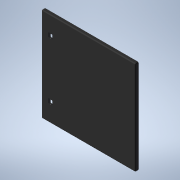
# Autodesk Inventor part: 155X_01_01(1)_P2
Saved by Autodesk Inventor 2021 (Build 250183000, 183)
## iProperties
Created: 2025-07-29
Part Number: 155X_01_01(1)_P2
Material: Generic
Catalog Web Link: www.cadenas.de
Description: AE 2.0 Einzeltuer-AE 2.0 Einzeltuer
Vendor: RITTAL
Document SubType Name: Modeling
Designer: psAdmin
Manufacturer: RITTAL
Mass: 530.122 g
Surface Area: 6232.6 cm^2
Volume: 530.122 cm^3
Density: 1 g/cm^3
Appearance: PSOLRGB-176-176-176
Category: PARTsolutions
Company: RITTAL
Title: 155X_01_01(1)_P2
Author: Cadenas PARTsolutions
Comments: AE 2.0 Einzeltuer
PSOL_IDENT_0: {$CADENAS_DATA/23d-libs/rittal/schaltschranksys/kompakt_schaltschr/parts_ae_2_0/einzeltuer_ae_2_0.pr
PSOL_IDENT_1: j},196 {VTYP=3D},{NB=155X_01_01(1)_P2},{LINA=155X_01_01(1)_P2},{NN=AE 2.0 Einzeltuer},{DATE=28.04.20
PSOL_IDENT_2: 25 21:11:31},{GEOMDATE=11.04.2025 11:21:47},{VERSION=},{LINEID=180},{WBVAR=DETAIL},{WBNUMERIC=DETAIL
PSOL_IDENT_3: }  {NB=155X_01_01(1)_P2},{LINA=155X_01_01(1)_P2},{KT=DUMMY},{BEST=155X},{DETAIL=1},{BEZ1=Neues Kompa
PSOL_IDENT_4: ktgehäuse},{BEZ2=Stahlblech},{BEZ3=eintürig},{B=500},{H=500},{VERS=1},{W=494},{W1=425},{W3=0},{HH=49
PSOL_IDENT_5: 4},{H1=375},{H2=440},{H4=58.0},{H5=300.000},{H6=350.000},{H7=350.000},{D=16.5},{ST=1.5},{R1=5.0},{GE
PSOL_IDENT_6: W=0},{CNSECLASS51=27-18-01-02},{CNSECLASS70=27-18-01-01},{CNSECLASS80=27-18-01-01},{CNSETIM40=EC0002
PSOL_IDENT_7: 61}
NB: 155X_01_01(1)_P2
NN: AE 2.0 Einzeltuer
NT: AE 2.0 Einzeltuer
NBSYN: $BEST._01_01($DETAIL.)_P2
LINA: 155X_01_01(1)_P2
CATALOG: Rittal
BEST: 155X
DETAIL: hoch
BEZ1: Neues Kompaktgehäuse
BEZ2: Stahlblech
BEZ3: eintürig
B: 500
H: 500
VERS: 1
W: 494
W1: 425
W3: 0
HH: 494
H1: 375
H2: 440
H4: 58
H5: 300
H6: 350
H7: 350
D: 16.5
ST: 1.5
R1: 5
GEW: 0
CNSECLASS70: 27-18-01-01
CNSECLASS80: 27-18-01-01
SUPPLIER: RITTAL
ARTICLENO: 155X_01_01(1)_P2
BOMINFO: 155X_01_01(1)_P2
CREATOR: CADENAS GmbH
Autodesk Inventor part; units mm, degrees
sketch "Sketch_1" plane through (0, 0, 0) normal (0, 1, 0) x (1, 0, 0)
  arc A0 (-247, 5) -> (-242, 0) centre (-242, 5) ccw
  line L0 (-242, 0) -> (242, 0)
  arc A1 (242, 0) -> (247, 5) centre (242, 5) ccw
  line L1 (247, 5) -> (247, 16.5)
  line L2 (247, 16.5) -> (245.5, 16.5)
  line L3 (245.5, 16.5) -> (245.5, 5)
  arc A2 (242, 1.5) -> (245.5, 5) centre (242, 5) ccw
  line L4 (242, 1.5) -> (-242, 1.5)
  arc A3 (-245.5, 5) -> (-242, 1.5) centre (-242, 5) ccw
  line L5 (-245.5, 5) -> (-245.5, 16.5)
  line L6 (-245.5, 16.5) -> (-247, 16.5)
  line L7 (-247, 16.5) -> (-247, 5)
  constraints: 16 end point, 8 point on circle, 4 centre point
extrude "Extrusion1" add sketch "Sketch_1" along normal mid plane 484
sketch "Sketch_3" plane through (0, 242, 0) normal (0, 1, 0) x (1, 0, 0)
  line L0 (242, 0) -> (242, 16.5)
  arc A0 (242, 1.5) -> (245.5, 5) centre (242, 5) ccw
  line L1 (245.5, 5) -> (245.5, 16.5)
  line L2 (245.5, 16.5) -> (247, 16.5)
  line L3 (247, 16.5) -> (247, 5)
  arc A1 (242, 0) -> (247, 5) centre (242, 5) ccw
  line L4 (242, 0) -> (242, 1.5)
  constraints: 10 end point, 4 point on circle, 2 centre point
revolve "Revolution1" add sketch "Sketch_3" angle 90 about axis through (242, 242, 0) along (0, 0, 1)
sketch "Sketch_4" plane through (0, 242, 0) normal (0, 1, 0) x (1, 0, 0)
  line L0 (-242, 16.5) -> (-242, 0)
  arc A0 (-247, 5) -> (-242, 0) centre (-242, 5) ccw
  line L1 (-247, 5) -> (-247, 16.5)
  line L2 (-247, 16.5) -> (-245.5, 16.5)
  line L3 (-245.5, 16.5) -> (-245.5, 5)
  arc A1 (-245.5, 5) -> (-242, 1.5) centre (-242, 5) ccw
  line L4 (-242, 1.5) -> (-242, 0)
  constraints: 10 end point, 4 point on circle, 2 centre point
revolve "Revolution2" add sketch "Sketch_4" angle 90 about axis through (-242, 242, -16.5) along (0, 0, -1)
sketch "Sketch_5" plane through (0, -242, 0) normal (0, 1, 0) x (1, 0, 0)
  line L0 (242, 0) -> (242, 16.5)
  arc A0 (242, 1.5) -> (245.5, 5) centre (242, 5) ccw
  line L1 (245.5, 5) -> (245.5, 16.5)
  line L2 (245.5, 16.5) -> (247, 16.5)
  line L3 (247, 16.5) -> (247, 5)
  arc A1 (242, 0) -> (247, 5) centre (242, 5) ccw
  line L4 (242, 0) -> (242, 1.5)
  constraints: 10 end point, 4 point on circle, 2 centre point
revolve "Revolution3" add sketch "Sketch_5" angle 90 about axis through (242, -242, 0) along (0, 0, -1)
sketch "Sketch_6" plane through (0, -242, 0) normal (0, 1, 0) x (1, 0, 0)
  line L0 (-242, 16.5) -> (-242, 0)
  arc A0 (-247, 5) -> (-242, 0) centre (-242, 5) ccw
  line L1 (-247, 5) -> (-247, 16.5)
  line L2 (-247, 16.5) -> (-245.5, 16.5)
  line L3 (-245.5, 16.5) -> (-245.5, 5)
  arc A1 (-245.5, 5) -> (-242, 1.5) centre (-242, 5) ccw
  line L4 (-242, 1.5) -> (-242, 0)
  constraints: 10 end point, 4 point on circle, 2 centre point
revolve "Revolution4" add sketch "Sketch_6" angle 90 about axis through (-242, -242, -16.5) along (0, 0, 1)
sketch "Sketch_2" plane through (0, 0, 0) normal (1, 0, 0) x (0, 0, -1)
  line L0 (0, 242) -> (0, -242)
  arc A0 (0, -242) -> (5, -247) centre (5, -242) ccw
  line L1 (5, -247) -> (16.5, -247)
  line L2 (16.5, -247) -> (16.5, -245.5)
  line L3 (16.5, -245.5) -> (5, -245.5)
  arc A1 (1.5, -242) -> (5, -245.5) centre (5, -242) ccw
  line L4 (1.5, -242) -> (1.5, 242)
  arc A2 (5, 245.5) -> (1.5, 242) centre (5, 242) ccw
  line L5 (5, 245.5) -> (16.5, 245.5)
  line L6 (16.5, 245.5) -> (16.5, 247)
  line L7 (16.5, 247) -> (5, 247)
  arc A3 (5, 247) -> (0, 242) centre (5, 242) ccw
  constraints: 16 end point, 8 point on circle, 4 centre point
extrude "Extrusion2" add sketch "Sketch_2" along normal mid plane 484
sketch "Sketch_44" plane through (231, 0, 0) normal (1, 0, 0) x (0, 0, -1)
  line L0 (1.5, -224.6934) -> (1.5, 224.6934)
  line L1 (1.5, 224.6934) -> (7.5, 224.6934)
  line L2 (7.5, 224.6934) -> (7, 208)
  line L3 (7, 208) -> (7, -208)
  line L4 (7, -208) -> (7.5, -224.6934)
  line L5 (7.5, -224.6934) -> (1.5, -224.6934)
  line L6 (1.5, -224.6934) -> (1.5, 224.6934)
  constraints: 14 end point
revolve "Revolution5" add sketch "Sketch_44" angle 180 mid plane about axis through (231, -224.6934, -1.5) along (0, 1, 0)
sketch "Sketch_45" plane through (0, 224.6934, 0) normal (0, 1, 0) x (1, 0, 0)
  line L0 (241, 7.5) -> (241, 1.5)
  line L1 (225, 1.5) -> (237, 1.5)
  arc A0 (237, 1.5) -> (225, 1.5) centre (231, 1.5) ccw
  constraints: 4 end point, 2 point on circle, 1 centre point
revolve "Revolution6" add sketch "Sketch_45" angle 39.715 about axis through (241, 224.6934, -7.5) along (0, 0, -1)
sketch "Sketch_47" plane through (0, 224.6934, 0) normal (0, 1, 0) x (1, 0, 0)
  line L0 (-241, 1.5) -> (-241, 7.5)
  line L1 (-237, 1.5) -> (-225, 1.5)
  arc A0 (-225, 1.5) -> (-237, 1.5) centre (-231, 1.5) ccw
  constraints: 4 end point, 2 point on circle, 1 centre point
revolve "Revolution7" add sketch "Sketch_47" angle 39.715 about axis through (-241, 224.6934, -1.5) along (0, 0, 1)
sketch "Sketch_46" plane through (241, 224.6934, 0) normal (-0.6389711, -0.7692308, 0) x (-0.7692308, 0.6389711, 0)
  line L0 (13, 6.6962) -> (13, 1.5)
  line L1 (13, 1.5) -> (4, 1.5)
  arc A0 (13, 6.6962) -> (4, 1.5) centre (10, 1.5) ccw
  line L2 (13, 6.6962) -> (13, 1.5)
  constraints: 6 end point, 2 point on circle, 1 centre point
revolve "Revolution8" add sketch "Sketch_46" angle 169.43 about axis through (231, 233, -6.6962) along (0, 0, 1)
sketch "Sketch_49" plane through (-241, 224.6934, 0) normal (-0.6389711, 0.7692308, 0) x (0.7692308, 0.6389711, 0)
  line L0 (13, 6.6962) -> (13, 1.5)
  line L1 (13, 1.5) -> (4, 1.5)
  arc A0 (13, 6.6962) -> (4, 1.5) centre (10, 1.5) ccw
  line L2 (13, 6.6962) -> (13, 1.5)
  constraints: 6 end point, 2 point on circle, 1 centre point
revolve "Revolution9" add sketch "Sketch_49" angle 169.43 about axis through (-231, 233, -6.6962) along (0, 0, -1)
sketch "Sketch_48" plane through (231, 233, 0) normal (-0.7692308, -0.6389711, 0) x (-0.6389711, 0.7692308, 0)
  line L0 (13, 7.5) -> (13, 1.5)
  line L1 (-3, 1.5) -> (9, 1.5)
  arc A0 (9, 1.5) -> (-3, 1.5) centre (3, 1.5) ccw
  constraints: 4 end point, 2 point on circle, 1 centre point
revolve "Revolution10" add sketch "Sketch_48" angle 39.715 about axis through (222.6934, 243, -7.5) along (0, 0, -1)
sketch "Sketch_50" plane through (-231, 233, 0) normal (-0.7692308, 0.6389711, 0) x (0.6389711, 0.7692308, 0)
  line L0 (13, 7.5) -> (13, 1.5)
  line L1 (-3, 1.5) -> (9, 1.5)
  arc A0 (9, 1.5) -> (-3, 1.5) centre (3, 1.5) ccw
  constraints: 4 end point, 2 point on circle, 1 centre point
revolve "Revolution11" add sketch "Sketch_50" angle 39.715 about axis through (-222.6934, 243, -7.5) along (0, 0, 1)
sketch "Sketch_51" plane through (-231, 0, 0) normal (1, 0, 0) x (0, 0, -1)
  line L0 (1.5, -224.6934) -> (1.5, 224.6934)
  line L1 (1.5, 224.6934) -> (7.5, 224.6934)
  line L2 (7.5, 224.6934) -> (7, 208)
  line L3 (7, 208) -> (7, -208)
  line L4 (7, -208) -> (7.5, -224.6934)
  line L5 (7.5, -224.6934) -> (1.5, -224.6934)
  line L6 (1.5, -224.6934) -> (1.5, 224.6934)
  constraints: 14 end point
revolve "Revolution12" add sketch "Sketch_51" angle 180 mid plane about axis through (-231, -224.6934, -1.5) along (0, 1, 0)
sketch "Sketch_52" plane through (0, -224.6934, 0) normal (0, 1, 0) x (1, 0, 0)
  line L0 (241, 7.5) -> (241, 1.5)
  line L1 (225, 1.5) -> (237, 1.5)
  arc A0 (237, 1.5) -> (225, 1.5) centre (231, 1.5) ccw
  constraints: 4 end point, 2 point on circle, 1 centre point
revolve "Revolution13" add sketch "Sketch_52" angle 39.715 about axis through (241, -224.6934, -7.5) along (0, 0, 1)
sketch "Sketch_53" plane through (0, -224.6934, 0) normal (0, 1, 0) x (1, 0, 0)
  line L0 (-241, 1.5) -> (-241, 7.5)
  line L1 (-237, 1.5) -> (-225, 1.5)
  arc A0 (-225, 1.5) -> (-237, 1.5) centre (-231, 1.5) ccw
  constraints: 4 end point, 2 point on circle, 1 centre point
revolve "Revolution14" add sketch "Sketch_53" angle 39.715 about axis through (-241, -224.6934, -1.5) along (0, 0, -1)
sketch "Sketch_54" plane through (241, -224.6934, 0) normal (0.6389711, -0.7692308, 0) x (-0.7692308, -0.6389711, 0)
  line L0 (13, 6.6962) -> (13, 1.5)
  line L1 (13, 1.5) -> (4, 1.5)
  arc A0 (13, 6.6962) -> (4, 1.5) centre (10, 1.5) ccw
  line L2 (13, 6.6962) -> (13, 1.5)
  constraints: 6 end point, 2 point on circle, 1 centre point
revolve "Revolution15" add sketch "Sketch_54" angle 169.43 about axis through (231, -233, -6.6962) along (0, 0, -1)
sketch "Sketch_55" plane through (231, -233, 0) normal (0.7692308, -0.6389711, 0) x (-0.6389711, -0.7692308, 0)
  line L0 (13, 7.5) -> (13, 1.5)
  line L1 (-3, 1.5) -> (9, 1.5)
  arc A0 (9, 1.5) -> (-3, 1.5) centre (3, 1.5) ccw
  constraints: 4 end point, 2 point on circle, 1 centre point
revolve "Revolution16" add sketch "Sketch_55" angle 39.715 about axis through (222.6934, -243, -7.5) along (0, 0, 1)
sketch "Sketch_56" plane through (-241, -224.6934, 0) normal (-0.6389711, -0.7692308, 0) x (-0.7692308, 0.6389711, 0)
  line L0 (-13, 1.5) -> (-13, 6.6962)
  arc A0 (-4, 1.5) -> (-13, 6.6962) centre (-10, 1.5) ccw
  line L1 (-4, 1.5) -> (-13, 1.5)
  line L2 (-13, 1.5) -> (-13, 6.6962)
  constraints: 6 end point, 2 point on circle, 1 centre point
revolve "Revolution17" add sketch "Sketch_56" angle 169.43 about axis through (-231, -233, -1.5) along (0, 0, 1)
sketch "Sketch_57" plane through (-231, -233, 0) normal (0.7692308, 0.6389711, 0) x (0.6389711, -0.7692308, 0)
  line L0 (13, 7.5) -> (13, 1.5)
  line L1 (-3, 1.5) -> (9, 1.5)
  arc A0 (9, 1.5) -> (-3, 1.5) centre (3, 1.5) ccw
  constraints: 4 end point, 2 point on circle, 1 centre point
revolve "Revolution18" add sketch "Sketch_57" angle 39.715 about axis through (-222.6934, -243, -7.5) along (0, 0, -1)
sketch "Sketch_58" plane through (0, 233, 0) normal (0, 1, 0) x (1, 0, 0)
  line L0 (222.6934, 1.5) -> (-222.6934, 1.5)
  line L1 (-222.6934, 1.5) -> (-222.6934, 7.5)
  line L2 (-222.6934, 7.5) -> (222.6934, 7.5)
  line L3 (222.6934, 7.5) -> (222.6934, 1.5)
  line L4 (222.6934, 1.5) -> (-222.6934, 1.5)
  constraints: 10 end point
revolve "Revolution19" add sketch "Sketch_58" angle 180 mid plane about axis through (222.6934, 233, -1.5) along (-1, 0, 0)
sketch "Sketch_59" plane through (0, -233, 0) normal (0, 1, 0) x (1, 0, 0)
  line L0 (222.6934, 1.5) -> (-222.6934, 1.5)
  line L1 (-222.6934, 1.5) -> (-222.6934, 7.5)
  line L2 (-222.6934, 7.5) -> (222.6934, 7.5)
  line L3 (222.6934, 7.5) -> (222.6934, 1.5)
  line L4 (222.6934, 1.5) -> (-222.6934, 1.5)
  constraints: 10 end point
revolve "Revolution20" add sketch "Sketch_59" angle 180 mid plane about axis through (222.6934, -233, -1.5) along (-1, 0, 0)
sketch "Sketch_7" plane through (0, -187.5, 0) normal (0, 1, 0) x (1, 0, 0)
  arc A0 (240.5, 14.6) -> (240.5, 6.4) centre (240.5, 10.5) ccw
  line L0 (240.5, 6.4) -> (245.5, 6.4)
  line L1 (245.5, 6.4) -> (245.5, 7.9)
  line L2 (245.5, 7.9) -> (240.5, 7.9)
  arc A1 (240.5, 13.1) -> (240.5, 7.9) centre (240.5, 10.5) ccw
  line L3 (240.5, 13.1) -> (245.5, 13.1)
  line L4 (245.5, 13.1) -> (245.5, 14.6)
  line L5 (245.5, 14.6) -> (240.5, 14.6)
  constraints: 12 end point, 4 point on circle, 2 centre point
extrude "Extrusion3" add sketch "Sketch_7" along normal mid plane 19.7
sketch "Sketch_8" plane through (0, 187.5, 0) normal (0, 1, 0) x (1, 0, 0)
  arc A0 (240.5, 14.6) -> (240.5, 6.4) centre (240.5, 10.5) ccw
  line L0 (240.5, 6.4) -> (245.5, 6.4)
  line L1 (245.5, 6.4) -> (245.5, 7.9)
  line L2 (245.5, 7.9) -> (240.5, 7.9)
  arc A1 (240.5, 13.1) -> (240.5, 7.9) centre (240.5, 10.5) ccw
  line L3 (240.5, 13.1) -> (245.5, 13.1)
  line L4 (245.5, 13.1) -> (245.5, 14.6)
  line L5 (245.5, 14.6) -> (240.5, 14.6)
  constraints: 12 end point, 4 point on circle, 2 centre point
extrude "Extrusion4" add sketch "Sketch_8" along normal mid plane 19.7
sketch "Sketch_11" plane through (0, 0, 0) normal (0, 1, 0) x (1, 0, 0)
  line L0 (204.5, 15.4) -> (204.5, 1.5)
  line L1 (204.5, 1.5) -> (205.3, 1.5)
  line L2 (205.3, 1.5) -> (205.3, 15.4)
  arc A0 (206.1, 16.2) -> (205.3, 15.4) centre (206.1, 15.4) ccw
  line L3 (206.1, 16.2) -> (218.4, 16.2)
  arc A1 (219.2, 15.4) -> (218.4, 16.2) centre (218.4, 15.4) ccw
  line L4 (219.2, 15.4) -> (219.2, 1.5)
  line L5 (219.2, 1.5) -> (220, 1.5)
  line L6 (220, 1.5) -> (220, 15.4)
  arc A2 (220, 15.4) -> (218.4, 17) centre (218.4, 15.4) ccw
  line L7 (218.4, 17) -> (206.1, 17)
  arc A3 (206.1, 17) -> (204.5, 15.4) centre (206.1, 15.4) ccw
  constraints: 16 end point, 8 point on circle, 4 centre point
extrude "Extrusion5" add sketch "Sketch_11" along normal mid plane 440
sketch "Sketch_12" plane through (0, 0, 0) normal (0, 1, 0) x (1, 0, 0)
  line L0 (-220.5, 15.4) -> (-220.5, 1.5)
  line L1 (-220.5, 1.5) -> (-219.7, 1.5)
  line L2 (-219.7, 1.5) -> (-219.7, 15.4)
  arc A0 (-218.9, 16.2) -> (-219.7, 15.4) centre (-218.9, 15.4) ccw
  line L3 (-218.9, 16.2) -> (-206.6, 16.2)
  arc A1 (-205.8, 15.4) -> (-206.6, 16.2) centre (-206.6, 15.4) ccw
  line L4 (-205.8, 15.4) -> (-205.8, 1.5)
  line L5 (-205.8, 1.5) -> (-205, 1.5)
  line L6 (-205, 1.5) -> (-205, 15.4)
  arc A2 (-205, 15.4) -> (-206.6, 17) centre (-206.6, 15.4) ccw
  line L7 (-206.6, 17) -> (-218.9, 17)
  arc A3 (-218.9, 17) -> (-220.5, 15.4) centre (-218.9, 15.4) ccw
  constraints: 16 end point, 8 point on circle, 4 centre point
extrude "Extrusion6" add sketch "Sketch_12" along normal mid plane 440
sketch "Sketch_13" plane through (212.25, 0, 0) normal (1, 0, 0) x (0, 0, -1)
  line L0 (14, 201) -> (14, 190.5)
  arc A0 (14, 190.5) -> (15, 189.5) centre (15, 190.5) ccw
  line L1 (15, 189.5) -> (18, 189.5)
  line L2 (18, 189.5) -> (18, -189.5)
  line L3 (18, -189.5) -> (15, -189.5)
  arc A1 (15, -189.5) -> (14, -190.5) centre (15, -190.5) ccw
  line L4 (14, -190.5) -> (14, -201)
  arc A2 (14, -201) -> (15, -202) centre (15, -201) ccw
  line L5 (15, -202) -> (22, -202)
  line L6 (22, -202) -> (22, 202)
  line L7 (22, 202) -> (15, 202)
  arc A3 (15, 202) -> (14, 201) centre (15, 201) ccw
  constraints: 16 end point, 8 point on circle, 4 centre point
extrude "Extrusion7" cut sketch "Sketch_13" along normal mid plane 15.5
sketch "Sketch_15" plane through (212.25, 0, 0) normal (1, 0, 0) x (0, 0, -1)
  line L0 (15, 175) -> (17, 175)
  line L1 (17, 175) -> (17, 171.5)
  line L2 (17, 171.5) -> (16.2, 171.5)
  line L3 (16.2, 171.5) -> (16.2, 171.7)
  arc A0 (16.2, 171.7) -> (15.95, 171.95) centre (15.95, 171.7) ccw
  line L4 (15.95, 171.95) -> (15, 171.95)
  line L5 (15, 171.95) -> (15, 175)
  line L6 (15, 175) -> (17, 175)
  constraints: 14 end point, 2 point on circle, 1 centre point
revolve "Revolution21" add sketch "Sketch_15" angle 360 about axis through (212.25, 175, -15) along (0, 0, 1)
sketch "Sketch_14" plane through (-212.75, 0, 0) normal (1, 0, 0) x (0, 0, -1)
  line L0 (14, 201) -> (14, 190.5)
  arc A0 (14, 190.5) -> (15, 189.5) centre (15, 190.5) ccw
  line L1 (15, 189.5) -> (18, 189.5)
  line L2 (18, 189.5) -> (18, -189.5)
  line L3 (18, -189.5) -> (15, -189.5)
  arc A1 (15, -189.5) -> (14, -190.5) centre (15, -190.5) ccw
  line L4 (14, -190.5) -> (14, -201)
  arc A2 (14, -201) -> (15, -202) centre (15, -201) ccw
  line L5 (15, -202) -> (22, -202)
  line L6 (22, -202) -> (22, 202)
  line L7 (22, 202) -> (15, 202)
  arc A3 (15, 202) -> (14, 201) centre (15, 201) ccw
  constraints: 16 end point, 8 point on circle, 4 centre point
extrude "Extrusion8" cut sketch "Sketch_14" along normal mid plane 15.5
pattern_linear "Rectangular Pattern1" count 15 spacing 25 along (0, -1, 0) of "Revolution21"
sketch "Sketch_17" plane through (212.25, 0, 0) normal (1, 0, 0) x (0, 0, -1)
  line L0 (15, 175) -> (17.5, 175)
  line L1 (17.5, 175) -> (17.5, 172)
  line L2 (17.5, 172) -> (17, 172)
  line L3 (17, 172) -> (17, 172.25)
  arc A0 (17, 172.25) -> (16.5, 172.75) centre (16.5, 172.25) ccw
  line L4 (16.5, 172.75) -> (15, 172.75)
  line L5 (15, 172.75) -> (15, 175)
  line L6 (15, 175) -> (17.5, 175)
  constraints: 14 end point, 2 point on circle, 1 centre point
revolve "Revolution22" cut sketch "Sketch_17" angle 360 about axis through (212.25, 175, -15) along (0, 0, 1)
pattern_linear "Rectangular Pattern2" count 15 spacing 25 along (0, -1, 0) of "Revolution22"
sketch "Sketch_19" plane through (-212.75, 0, 0) normal (1, 0, 0) x (0, 0, -1)
  line L0 (15, 175) -> (17, 175)
  line L1 (17, 175) -> (17, 171.5)
  line L2 (17, 171.5) -> (16.2, 171.5)
  line L3 (16.2, 171.5) -> (16.2, 171.7)
  arc A0 (16.2, 171.7) -> (15.95, 171.95) centre (15.95, 171.7) ccw
  line L4 (15.95, 171.95) -> (15, 171.95)
  line L5 (15, 171.95) -> (15, 175)
  line L6 (15, 175) -> (17, 175)
  constraints: 14 end point, 2 point on circle, 1 centre point
revolve "Revolution23" add sketch "Sketch_19" angle 360 about axis through (-212.75, 175, -15) along (0, 0, 1)
pattern_linear "Rectangular Pattern3" count 15 spacing 25 along (0, -1, 0) of "Revolution23"
sketch "Sketch_21" plane through (-212.75, 0, 0) normal (1, 0, 0) x (0, 0, -1)
  line L0 (15, 175) -> (17.5, 175)
  line L1 (17.5, 175) -> (17.5, 172)
  line L2 (17.5, 172) -> (17, 172)
  line L3 (17, 172) -> (17, 172.25)
  arc A0 (17, 172.25) -> (16.5, 172.75) centre (16.5, 172.25) ccw
  line L4 (16.5, 172.75) -> (15, 172.75)
  line L5 (15, 172.75) -> (15, 175)
  line L6 (15, 175) -> (17.5, 175)
  constraints: 14 end point, 2 point on circle, 1 centre point
revolve "Revolution24" cut sketch "Sketch_21" angle 360 about axis through (-212.75, 175, -15) along (0, 0, 1)
pattern_linear "Rectangular Pattern4" count 15 spacing 25 along (0, -1, 0) of "Revolution24"
sketch "Sketch_23" plane through (0, 0, -17) normal (0, 0, 1) x (1, 0, 0)
  line L0 (210.25, 156.25) -> (214.25, 156.25)
  line L1 (214.25, 156.25) -> (214.25, 168.75)
  line L2 (214.25, 168.75) -> (210.25, 168.75)
  line L3 (210.25, 168.75) -> (210.25, 156.25)
  constraints: 8 end point
extrude "Extrusion9" cut sketch "Sketch_23" along normal blind 0.8
pattern_linear "Rectangular Pattern5" count 14 spacing 25 along (0, -1, 0) of "Extrusion9"
sketch "Sketch_25" plane through (0, 0, -17) normal (0, 0, 1) x (1, 0, 0)
  line L0 (-214.75, 156.25) -> (-210.75, 156.25)
  line L1 (-210.75, 156.25) -> (-210.75, 168.75)
  line L2 (-210.75, 168.75) -> (-214.75, 168.75)
  line L3 (-214.75, 168.75) -> (-214.75, 156.25)
  constraints: 8 end point
extrude "Extrusion10" cut sketch "Sketch_25" along normal blind 0.8
pattern_linear "Rectangular Pattern6" count 14 spacing 25 along (0, -1, 0) of "Extrusion10"
sketch "Sketch_27" plane through (0, 0, -17) normal (0, 0, 1) x (1, 0, 0)
  line L0 (-215.6, 167) -> (-215.6, 133)
  arc A0 (-215.6, 133) -> (-212.6, 130) centre (-212.6, 133) ccw
  line L1 (-212.6, 130) -> (-200.6, 130)
  line L2 (-200.6, 130) -> (-200.6, 170)
  line L3 (-200.6, 170) -> (-212.6, 170)
  arc A1 (-212.6, 170) -> (-215.6, 167) centre (-212.6, 167) ccw
  constraints: 8 end point, 4 point on circle, 2 centre point
extrude "Extrusion11" cut sketch "Sketch_27" along normal blind 15.5
sketch "Sketch_28" plane through (0, 0, -17) normal (0, 0, 1) x (1, 0, 0)
  line L0 (-215.6, -133) -> (-215.6, -167)
  arc A0 (-215.6, -167) -> (-212.6, -170) centre (-212.6, -167) ccw
  line L1 (-212.6, -170) -> (-200.6, -170)
  line L2 (-200.6, -170) -> (-200.6, -130)
  line L3 (-200.6, -130) -> (-212.6, -130)
  arc A1 (-212.6, -130) -> (-215.6, -133) centre (-212.6, -133) ccw
  constraints: 8 end point, 4 point on circle, 2 centre point
extrude "Extrusion12" cut sketch "Sketch_28" along normal blind 15.5
sketch "Sketch_29" plane through (0, 0, -17) normal (0, 0, 1) x (1, 0, 0)
  line L0 (207, 202) -> (207, 201)
  line L1 (207, 201) -> (217.5, 201)
  line L2 (217.5, 201) -> (217.5, 202)
  arc A0 (216.5, 203) -> (217.5, 202) centre (217.5, 203) ccw
  line L3 (216.5, 203) -> (216.5, 210.5)
  arc A1 (216.5, 210.5) -> (208, 210.5) centre (212.25, 210.5) ccw
  line L4 (208, 210.5) -> (208, 203)
  arc A2 (207, 202) -> (208, 203) centre (207, 203) ccw
  constraints: 10 end point, 6 point on circle, 3 centre point
extrude "Extrusion13" cut sketch "Sketch_29" along normal blind 0.8
sketch "Sketch_30" plane through (0, 0, -17) normal (0, 0, 1) x (1, 0, 0)
  arc A0 (208, -203) -> (207, -202) centre (207, -203) ccw
  line L0 (208, -203) -> (208, -210.5)
  arc A1 (208, -210.5) -> (216.5, -210.5) centre (212.25, -210.5) ccw
  line L1 (216.5, -210.5) -> (216.5, -203)
  arc A2 (217.5, -202) -> (216.5, -203) centre (217.5, -203) ccw
  line L2 (217.5, -202) -> (217.5, -201)
  line L3 (217.5, -201) -> (207, -201)
  line L4 (207, -201) -> (207, -202)
  constraints: 10 end point, 6 point on circle, 3 centre point
extrude "Extrusion14" cut sketch "Sketch_30" along normal blind 0.8
sketch "Sketch_31" plane through (0, 0, -17) normal (0, 0, 1) x (1, 0, 0)
  line L0 (-218, 202) -> (-218, 201)
  line L1 (-218, 201) -> (-207.5, 201)
  line L2 (-207.5, 201) -> (-207.5, 202)
  arc A0 (-208.5, 203) -> (-207.5, 202) centre (-207.5, 203) ccw
  line L3 (-208.5, 203) -> (-208.5, 210.5)
  arc A1 (-208.5, 210.5) -> (-217, 210.5) centre (-212.75, 210.5) ccw
  line L4 (-217, 210.5) -> (-217, 203)
  arc A2 (-218, 202) -> (-217, 203) centre (-218, 203) ccw
  constraints: 10 end point, 6 point on circle, 3 centre point
extrude "Extrusion15" cut sketch "Sketch_31" along normal blind 0.8
sketch "Sketch_32" plane through (0, 0, -17) normal (0, 0, 1) x (1, 0, 0)
  arc A0 (-217, -203) -> (-218, -202) centre (-218, -203) ccw
  line L0 (-217, -203) -> (-217, -210.5)
  arc A1 (-217, -210.5) -> (-208.5, -210.5) centre (-212.75, -210.5) ccw
  line L1 (-208.5, -210.5) -> (-208.5, -203)
  arc A2 (-207.5, -202) -> (-208.5, -203) centre (-207.5, -203) ccw
  line L2 (-207.5, -202) -> (-207.5, -201)
  line L3 (-207.5, -201) -> (-218, -201)
  line L4 (-218, -201) -> (-218, -202)
  constraints: 10 end point, 6 point on circle, 3 centre point
extrude "Extrusion16" cut sketch "Sketch_32" along normal blind 0.8
sketch "Sketch_33" plane through (0, 0, 0) normal (0, 0, 1) x (1, 0, 0)
  line L0 (-211.15, 160.65) -> (-211.15, 139.35)
  arc A0 (-211.15, 139.35) -> (-210.65, 138.85) centre (-210.65, 139.35) ccw
  line L1 (-210.65, 138.85) -> (-189.35, 138.85)
  arc A1 (-189.35, 138.85) -> (-188.85, 139.35) centre (-189.35, 139.35) ccw
  line L2 (-188.85, 139.35) -> (-188.85, 160.65)
  arc A2 (-188.85, 160.65) -> (-189.35, 161.15) centre (-189.35, 160.65) ccw
  line L3 (-189.35, 161.15) -> (-202.65, 161.15)
  arc A3 (-203.15, 161.65) -> (-202.65, 161.15) centre (-202.65, 161.65) ccw
  line L4 (-203.15, 161.65) -> (-203.15, 162.15)
  arc A4 (-203.15, 162.15) -> (-203.65, 162.65) centre (-203.65, 162.15) ccw
  line L5 (-203.65, 162.65) -> (-208.65, 162.65)
  arc A5 (-208.65, 162.65) -> (-209.15, 162.15) centre (-208.65, 162.15) ccw
  line L6 (-209.15, 162.15) -> (-209.15, 161.65)
  arc A6 (-209.65, 161.15) -> (-209.15, 161.65) centre (-209.65, 161.65) ccw
  line L7 (-209.65, 161.15) -> (-210.65, 161.15)
  arc A7 (-210.65, 161.15) -> (-211.15, 160.65) centre (-210.65, 160.65) ccw
  constraints: 16 end point, 16 point on circle, 8 centre point
extrude "Extrusion17" cut sketch "Sketch_33" against normal blind 1.5
sketch "Sketch_34" plane through (0, 0, 0) normal (0, 0, 1) x (1, 0, 0)
  line L0 (-211.15, -139.35) -> (-211.15, -160.65)
  arc A0 (-211.15, -160.65) -> (-210.65, -161.15) centre (-210.65, -160.65) ccw
  line L1 (-210.65, -161.15) -> (-189.35, -161.15)
  arc A1 (-189.35, -161.15) -> (-188.85, -160.65) centre (-189.35, -160.65) ccw
  line L2 (-188.85, -160.65) -> (-188.85, -139.35)
  arc A2 (-188.85, -139.35) -> (-189.35, -138.85) centre (-189.35, -139.35) ccw
  line L3 (-189.35, -138.85) -> (-202.65, -138.85)
  arc A3 (-203.15, -138.35) -> (-202.65, -138.85) centre (-202.65, -138.35) ccw
  line L4 (-203.15, -138.35) -> (-203.15, -137.85)
  arc A4 (-203.15, -137.85) -> (-203.65, -137.35) centre (-203.65, -137.85) ccw
  line L5 (-203.65, -137.35) -> (-208.65, -137.35)
  arc A5 (-208.65, -137.35) -> (-209.15, -137.85) centre (-208.65, -137.85) ccw
  line L6 (-209.15, -137.85) -> (-209.15, -138.35)
  arc A6 (-209.65, -138.85) -> (-209.15, -138.35) centre (-209.65, -138.35) ccw
  line L7 (-209.65, -138.85) -> (-210.65, -138.85)
  arc A7 (-210.65, -138.85) -> (-211.15, -139.35) centre (-210.65, -139.35) ccw
  constraints: 16 end point, 16 point on circle, 8 centre point
extrude "Extrusion18" cut sketch "Sketch_34" against normal blind 1.5
ref_plane "ET_XY" through (240.5, -187.5, -10.5) normal (0, 1, 0) x (1, 0, 0)
ref_plane "ET_YZ" through (240.5, -187.5, -10.5) normal (1, 0, 0) x (0, 0, -1)
ref_plane "ET_ZX" through (240.5, -187.5, -10.5) normal (0, 0, -1) x (0, 1, 0)
ref_plane "SC_XY" through (245.5, 0, 0) normal (0, 0, -1) x (1, 0, 0)
ref_plane "SC_YZ" through (245.5, 0, 0) normal (1, 0, 0) x (0, -1, 0)
ref_plane "SC_ZX" through (245.5, 0, 0) normal (0, -1, 0) x (0, 0, -1)
ref_plane "VV1_XY" through (-200, 150, 0) normal (0, 0, -1) x (1, 0, 0)
ref_plane "VV1_YZ" through (-200, 150, 0) normal (1, 0, 0) x (0, -1, 0)
ref_plane "VV1_ZX" through (-200, 150, 0) normal (0, -1, 0) x (0, 0, -1)
ref_plane "VV2_XY" through (-200, -150, 0) normal (0, 0, -1) x (1, 0, 0)
ref_plane "VV2_YZ" through (-200, -150, 0) normal (1, 0, 0) x (0, -1, 0)
ref_plane "VV2_ZX" through (-200, -150, 0) normal (0, -1, 0) x (0, 0, -1)
ref_plane "to_Auflaufelement_XY" through (-212.75, -210.5, -17) normal (0, 0, 1) x (1, 0, 0)
ref_plane "to_Auflaufelement_YZ" through (-212.75, -210.5, -17) normal (1, 0, 0) x (0, 1, 0)
ref_plane "to_Auflaufelement_ZX" through (-212.75, -210.5, -17) normal (0, 1, 0) x (0, 0, 1)
body "Solid1"
